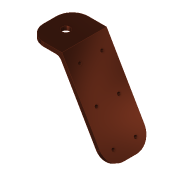
# Autodesk Inventor part: matrix_holder
Saved by Autodesk Inventor 2019 (Build 230136000, 136)
## iProperties
Created: 2019-02-25
Part Number: matrix_holder
Material: Generic
Document SubType Name: Modeling
Designer: Brian
Density: 1 g/cm^3
Appearance: Copper - Polished
Author: Brian
Autodesk Inventor part; units mm, degrees
ref_plane "YZ Plane" through (0, 0, 0) normal (1, 0, 0) x (0, 1, 0)
ref_plane "XZ Plane" through (0, 0, 0) normal (0, 1, 0) x (-1, 0, 0)
ref_plane "XY Plane" through (0, 0, 0) normal (0, 0, 1) x (1, 0, 0)
sketch "Sketch1" plane through (0, 0, 0) normal (0, 0, 1) x (1, 0, 0)
  line L0 (13.3846, -4.4923) -> (-12.0154, -4.4923)
  line L1 (-12.0154, -1.3173) -> (-12.0154, -4.4923)
  line L2 (13.3846, -4.4923) -> (84.5046, -4.4923) construction
  line L3 (13.3846, -4.4923) -> (84.5046, -4.4923) construction
  line L4 (13.3846, -4.4923) -> (84.5046, -4.4923) construction
  line L5 (13.3846, -4.4923) -> (48.9446, -66.084)
  line L6 (13.3846, -4.4923) -> (84.5046, -4.4923) construction
  line L7 (48.9446, -66.084) -> (51.6943, -64.4965)
  line L8 (-12.0154, -1.3173) -> (15.2177, -1.3173)
  line L9 (51.6943, -64.4965) -> (15.2177, -1.3173)
  dimension "d13" = 3.175
  dimension "d30" = 71.12
  dimension "d31" = 60
  dimension "d32" = 3.175
  constraints: 20 end point, 5 horizontal, 2 parallel, 2 perpendicular, 1 equal length
  measures "d13" distance of L1.start L0.end
  measures "d30" distance of L0.start L5.end
  measures "d31" angle of L5 L6
  measures "d32" distance of L5.end L7.end
extrude "Extrusion1" add sketch "Sketch1" along normal blind 35.56
sketch "Sketch2" plane through (-12.0154, -1.3173, 0) normal (0, 1, 0) x (1, 0, 0)
  line L0 (0, 0) -> (27.2331, 0) projected
  line L1 (0, 0) -> (0, -35.56) projected
  point P0 (12.0154, 0)
  point P1 (12.7, -17.78)
  dimension "d45" = 17.78
  dimension "d46" = 12.7
  measures "d45" distance from line of L0 point (12.7, -17.78)
  measures "d46" distance from line of L1 point (12.7, -17.78)
hole "Hole1" at (0.6846, -1.3173, 17.78) direction (0, -1, 0) diameter 6.604 depth 3.175 tip angle 118
sketch "Sketch3" plane through (15.2177, -1.3173, 35.56) normal (0.866, 0.5, 0) x (0, 0, -1)
  line L0 (35.56, -72.9531) -> (0, -72.9531) projected
  line L1 (35.56, 0) -> (35.56, -72.9531) projected
  point P0 (35.56, 8.7496)
  point P1 (26.67, -64.0631)
  dimension "d47" = 8.89
  dimension "d48" = 8.89
  measures "d47" distance from line of L0 point (26.67, -64.063)
  measures "d48" distance from line of L1 point (26.67, -64.063)
hole "Hole2" at (47.2493, -56.7975, 8.89) direction (-0.866, -0.5, 0) diameter 2.54 depth 3.175 tip angle 118
sketch "Sketch4" plane through (15.2177, -1.3173, 35.56) normal (0.866, 0.5, 0) x (0, 0, -1)
  line L0 (0, -72.9531) -> (0, 0) projected
  line L1 (35.56, -72.9531) -> (0, -72.9531) projected
  point P0 (35.56, 8.7496)
  point P1 (8.89, -64.0631)
  dimension "d56" = 8.89
  dimension "d57" = 8.89
  measures "d56" distance from line of L0 point (8.89, -64.063)
  measures "d57" distance from line of L1 point (8.89, -64.063)
hole "Hole3" at (47.2493, -56.7975, 26.67) direction (-0.866, -0.5, 0) diameter 2.54 depth 3.175 tip angle 118
sketch "Sketch5" plane through (15.2177, -1.3173, 35.56) normal (0.866, 0.5, 0) x (0, 0, -1)
  line L0 (0, -72.9531) -> (0, 0) projected
  line L1 (35.56, -72.9531) -> (0, -72.9531) projected
  point P0 (35.56, 8.7496)
  point P1 (8.89, -37.3931)
  dimension "d65" = 8.89
  dimension "d66" = 35.56
  measures "d65" distance from line of L0 point (8.89, -37.393)
  measures "d66" distance from line of L1 point (8.89, -37.393)
hole "Hole4" at (33.9143, -33.7006, 26.67) direction (-0.866, -0.5, 0) diameter 2.54 depth 3.175 tip angle 118
sketch "Sketch6" plane through (15.2177, -1.3173, 35.56) normal (0.866, 0.5, 0) x (0, 0, -1)
  line L0 (35.56, 0) -> (35.56, -72.9531) projected
  line L1 (35.56, -72.9531) -> (0, -72.9531) projected
  point P0 (35.56, 8.7496)
  point P1 (26.67, -37.3931)
  dimension "d74" = 8.89
  dimension "d75" = 35.56
  measures "d74" distance from line of L0 point (26.67, -37.393)
  measures "d75" distance from line of L1 point (26.67, -37.393)
hole "Hole5" at (33.9143, -33.7006, 8.89) direction (-0.866, -0.5, 0) diameter 2.54 depth 3.175 tip angle 118
sketch "Sketch7" plane through (15.2177, -1.3173, 35.56) normal (0.866, 0.5, 0) x (0, 0, -1)
  line L0 (35.56, 0) -> (35.56, -72.9531) projected
  line L1 (35.56, 0) -> (0, 0) projected
  circle A0 centre (26.67, -37.3931) radius 1.27 projected
  point P0 (35.56, 8.7496)
  point P1 (26.67, -10.7231)
  dimension "d83" = 8.89
  dimension "d101" = 26.67
  measures "d83" distance from line of L0 point (26.67, -10.723)
  measures "d101" distance of A0.centre point (26.67, -10.723)
hole "Hole6" at (20.5793, -10.6037, 8.89) direction (-0.866, -0.5, 0) diameter 2.54 depth 3.175 tip angle 118
sketch "Sketch8" plane through (15.2177, -1.3173, 35.56) normal (0.866, 0.5, 0) x (0, 0, -1)
  line L0 (35.56, 0) -> (0, 0) projected
  line L1 (0, -72.9531) -> (0, 0) projected
  circle A0 centre (8.89, -37.3931) radius 1.27 projected
  point P0 (35.56, 8.7496)
  point P1 (8.89, -10.7231)
  dimension "d93" = 8.89
  dimension "d102" = 26.67
  measures "d93" distance from line of L1 point (8.89, -10.723)
  measures "d102" distance of A0.centre point (8.89, -10.723)
hole "Hole7" at (20.5793, -10.6037, 26.67) direction (-0.866, -0.5, 0) diameter 2.54 depth 3.175 tip angle 118
fillet "Fillet1" radius 12.7 1 edges at (50.3194, -65.2902, 0)
fillet "Fillet2" radius 12.7 1 edges at (50.3194, -65.2902, 35.56)
fillet "Fillet3" radius 12.7 1 edges at (-12.0154, -2.9048, 35.56)
fillet "Fillet4" radius 12.7 1 edges at (-12.0154, -2.9048, 0)
fillet "Fillet5" radius 5.08 1 edges at (13.3846, -4.4923, 17.78)
body "Solid1"
